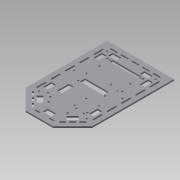
# Autodesk Inventor part: base kepala
Saved by Autodesk Inventor 2015 SP1 (Build 190203100, 203)
## iProperties
Created: 2015-02-14
Part Number: base kepala
Material: Generic
Document SubType Name: Modeling
Designer: Rafi Kurnia Putra
Density: 1 g/cm^3
Appearance: Default
Author: Rafi Kurnia Putra
Autodesk Inventor part; units mm, degrees
ref_plane "YZ Plane" through (0, 0, 0) normal (1, 0, 0) x (0, 1, 0)
ref_plane "XZ Plane" through (0, 0, 0) normal (0, 1, 0) x (-1, 0, 0)
ref_plane "XY Plane" through (0, 0, 0) normal (0, 0, 1) x (1, 0, 0)
sketch "Sketch1" plane through (0, 0, 0) normal (0, 1, 0) x (-1, 0, 0)
  line L0 (-8.75, -88.3884) -> (8.75, -88.3884)
  line L1 (-8.75, -78.3884) -> (-8.75, -88.3884)
  line L2 (8.75, -78.3884) -> (-8.75, -78.3884)
  line L3 (8.75, -88.3884) -> (8.75, -78.3884)
  line L4 (24.6113, -71.8184) -> (31.6823, -78.8894)
  line L5 (31.6823, -78.8894) -> (44.0567, -66.5151)
  line L6 (36.9856, -59.444) -> (24.6113, -71.8184)
  line L7 (44.0567, -66.5151) -> (36.9856, -59.444)
  line L8 (43.5557, -43.5826) -> (53.5557, -43.5826)
  line L9 (43.5557, -26.0826) -> (43.5557, -43.5826)
  line L10 (53.5557, -26.0826) -> (43.5557, -26.0826)
  line L11 (53.5557, -43.5826) -> (53.5557, -26.0826)
  line L12 (43.556, 62.6674) -> (53.556, 62.6674)
  line L13 (53.556, 62.6674) -> (53.556, 80.1674)
  line L14 (43.556, 80.1674) -> (43.556, 62.6674)
  line L15 (53.556, 80.1674) -> (43.556, 80.1674)
  line L16 (42.0848, 81.6386) -> (42.0848, 91.6386)
  line L17 (24.5848, 81.6386) -> (42.0848, 81.6386)
  line L18 (42.0848, 91.6386) -> (24.5848, 91.6386)
  line L19 (24.5848, 91.6386) -> (24.5848, 81.6386)
  line L20 (-24.5848, 81.6386) -> (-24.5848, 91.6386)
  line L21 (-42.0848, 81.6386) -> (-24.5848, 81.6386)
  line L22 (-42.0848, 91.6386) -> (-42.0848, 81.6386)
  line L23 (-24.5848, 91.6386) -> (-42.0848, 91.6386)
  line L24 (-53.556, 80.1674) -> (-53.556, 62.6674)
  line L25 (-43.556, 80.1674) -> (-53.556, 80.1674)
  line L26 (-43.556, 62.6674) -> (-43.556, 80.1674)
  line L27 (-53.556, 62.6674) -> (-43.556, 62.6674)
  line L28 (-43.5557, -26.0826) -> (-53.5557, -26.0826)
  line L29 (-43.5557, -43.5826) -> (-43.5557, -26.0826)
  line L30 (-53.5557, -43.5826) -> (-43.5557, -43.5826)
  line L31 (-53.5557, -26.0826) -> (-53.5557, -43.5826)
  line L32 (-32, -10.9442) -> (-32, -35.1896)
  line L33 (-22.2, -10.9442) -> (-32, -10.9442)
  line L34 (-22.2, -35.1896) -> (-22.2, -10.9442)
  line L35 (-32, -35.1896) -> (-22.2, -35.1896)
  line L36 (-31.6827, -78.8894) -> (-24.6116, -71.8184)
  line L37 (-44.057, -66.5151) -> (-31.6827, -78.8894)
  line L38 (-36.986, -59.444) -> (-44.057, -66.5151)
  line L39 (-24.6116, -71.8184) -> (-36.986, -59.444)
  line L40 (-24.5, 4.9331) -> (24.5, 4.9331)
  line L41 (24.5, 15.9376) -> (-24.5, 15.9376)
  line L42 (-24.5, 15.9376) -> (-24.5, 4.9331)
  line L43 (24.5, 4.9331) -> (24.5, 15.9376)
  circle A0 centre (-50.5965, 18.9376) radius 1.75
  circle A1 centre (-50.5965, 88.6786) radius 1.75
  circle A2 centre (-37.593, 75.6756) radius 1.75
  circle A3 centre (-32.8575, 75.4371) radius 1.75
  circle A4 centre (-32.4355, 53.6756) radius 1.75
  circle A5 centre (-32.442, 26.7171) radius 1.5
  circle A6 centre (14, 31.4596) radius 1.75
  circle A7 centre (-28, 4.9331) radius 1.75
  circle A8 centre (-49.906, -55.5042) radius 1.75
  circle A9 centre (-37.593, -48.9392) radius 1.75
  circle A10 centre (-27.94, -53.8096) radius 1.75
  circle A11 centre (-20, -65.0669) radius 1.75
  circle A12 centre (20, -65.0669) radius 1.75
  circle A13 centre (20.32, -47.4596) radius 1.75
  circle A14 centre (13.2193, -43.7996) radius 1.75
  circle A15 centre (13.2193, -19.3896) radius 1.75
  circle A16 centre (37.593, -48.9392) radius 1.75
  circle A17 centre (39.7053, -43.7996) radius 1.75
  circle A18 centre (49.9057, -55.5042) radius 1.75
  circle A19 centre (39.7053, -19.3896) radius 1.75
  circle A20 centre (28, 4.9331) radius 1.75
  circle A21 centre (32.442, 26.7171) radius 1.5
  circle A22 centre (38, 31.4596) radius 1.75
  circle A23 centre (50.5965, 18.9376) radius 1.75
  circle A24 centre (32.4485, 53.6756) radius 1.75
  circle A25 centre (32.8575, 75.4371) radius 1.75
  circle A26 centre (37.593, 75.6756) radius 1.75
  circle A27 centre (50.5965, 88.6786) radius 1.75
  line L44 (29.3575, 78.4256) -> (-29.3575, 78.4256)
  line L45 (29.3575, 72.4486) -> (29.3575, 78.4256)
  line L46 (-29.3575, 72.4486) -> (29.3575, 72.4486)
  line L47 (-29.3575, 78.4256) -> (-29.3575, 72.4486)
  line L48 (-5, -92.238) -> (5, -92.238)
  line L49 (5, -92.238) -> (5, -95.238)
  line L50 (5, -95.238) -> (-5, -95.238)
  line L51 (-5, -95.238) -> (-5, -92.238)
  line L52 (-5, -92.238) -> (5, -95.238) construction
  line L53 (5, -92.238) -> (-5, -95.238) construction
  line L54 (0, 0) -> (10, 0) construction
  line L55 (0, 0) -> (0, -10.9442) construction
  line L56 (10, -92.238) -> (20, -92.238)
  line L57 (20, -92.238) -> (20, -95.238)
  line L58 (20, -95.238) -> (10, -95.238)
  line L59 (10, -95.238) -> (10, -92.238)
  line L60 (10, -92.238) -> (20, -95.238) construction
  line L61 (20, -92.238) -> (10, -95.238) construction
  line L62 (-20, -92.238) -> (-10, -92.238)
  line L63 (-10, -92.238) -> (-10, -95.238)
  line L64 (-10, -95.238) -> (-20, -95.238)
  line L65 (-20, -95.238) -> (-20, -92.238)
  line L66 (-20, -92.238) -> (-10, -95.238) construction
  line L67 (-10, -92.238) -> (-20, -95.238) construction
  line L68 (-5, -92.238) -> (5, -92.238)
  line L69 (5, -92.238) -> (5, -95.238)
  line L70 (5, -95.238) -> (-5, -95.238)
  line L71 (-5, -95.238) -> (-5, -92.238)
  line L72 (-5, -92.238) -> (5, -95.238) construction
  line L73 (5, -92.238) -> (-5, -95.238) construction
  line L74 (39.1777, -81.0815) -> (46.2487, -74.0104)
  line L75 (46.2487, -74.0104) -> (44.1274, -71.8891)
  line L76 (44.1274, -71.8891) -> (37.0563, -78.9601)
  line L77 (37.0563, -78.9601) -> (39.1777, -81.0815)
  line L78 (39.1777, -81.0815) -> (44.1274, -71.8891) construction
  line L79 (46.2487, -74.0104) -> (37.0563, -78.9601) construction
  line L80 (0, 0) -> (-7.0711, -7.0711) construction
  line L81 (0, 0) -> (10, 0) construction
  line L82 (0, 0) -> (7.0711, -7.0711) construction
  line L83 (0, 0) -> (10, 0) construction
  line L84 (28.5711, -91.6881) -> (35.6421, -84.617)
  line L85 (35.6421, -84.617) -> (33.5208, -82.4957)
  line L86 (33.5208, -82.4957) -> (26.4497, -89.5667)
  line L87 (26.4497, -89.5667) -> (28.5711, -91.6881)
  line L88 (28.5711, -91.6881) -> (33.5208, -82.4957) construction
  line L89 (35.6421, -84.617) -> (26.4497, -89.5667) construction
  line L90 (49.7843, -70.4749) -> (56.8553, -63.4038)
  line L91 (56.8553, -63.4038) -> (54.734, -61.2825)
  line L92 (54.734, -61.2825) -> (47.6629, -68.3535)
  line L93 (47.6629, -68.3535) -> (49.7843, -70.4749)
  line L94 (49.7843, -70.4749) -> (54.734, -61.2825) construction
  line L95 (56.8553, -63.4038) -> (47.6629, -68.3535) construction
  line L96 (39.1777, -81.0815) -> (46.2487, -74.0104)
  line L97 (46.2487, -74.0104) -> (44.1274, -71.8891)
  line L98 (44.1274, -71.8891) -> (37.0563, -78.9601)
  line L99 (37.0563, -78.9601) -> (39.1777, -81.0815)
  line L100 (39.1777, -81.0815) -> (44.1274, -71.8891) construction
  line L101 (46.2487, -74.0104) -> (37.0563, -78.9601) construction
  line L102 (60.406, 8.4174) -> (57.406, 8.4174)
  line L103 (57.406, 8.4174) -> (57.406, 28.4174)
  line L104 (57.406, 28.4174) -> (60.406, 28.4174)
  line L105 (60.406, 28.4174) -> (60.406, 8.4174)
  line L106 (60.406, 8.4174) -> (57.406, 28.4174) construction
  line L107 (57.406, 8.4174) -> (60.406, 28.4174) construction
  line L108 (60.406, -21.5826) -> (57.406, -21.5826)
  line L109 (57.406, -21.5826) -> (57.406, -1.5826)
  line L110 (57.406, -1.5826) -> (60.406, -1.5826)
  line L111 (60.406, -1.5826) -> (60.406, -21.5826)
  line L112 (60.406, -21.5826) -> (57.406, -1.5826) construction
  line L113 (57.406, -21.5826) -> (60.406, -1.5826) construction
  line L114 (60.406, -51.5826) -> (57.406, -51.5826)
  line L115 (57.406, -51.5826) -> (57.406, -31.5826)
  line L116 (57.406, -31.5826) -> (60.406, -31.5826)
  line L117 (60.406, -31.5826) -> (60.406, -51.5826)
  line L118 (60.406, -51.5826) -> (57.406, -31.5826) construction
  line L119 (57.406, -51.5826) -> (60.406, -31.5826) construction
  line L120 (60.406, 38.4174) -> (57.406, 38.4174)
  line L121 (57.406, 38.4174) -> (57.406, 58.4174)
  line L122 (57.406, 58.4174) -> (60.406, 58.4174)
  line L123 (60.406, 58.4174) -> (60.406, 38.4174)
  line L124 (60.406, 38.4174) -> (57.406, 58.4174) construction
  line L125 (57.406, 38.4174) -> (60.406, 58.4174) construction
  line L126 (60.406, 8.4174) -> (57.406, 8.4174)
  line L127 (57.406, 8.4174) -> (57.406, 28.4174)
  line L128 (57.406, 28.4174) -> (60.406, 28.4174)
  line L129 (60.406, 28.4174) -> (60.406, 8.4174)
  line L130 (60.406, 8.4174) -> (57.406, 28.4174) construction
  line L131 (57.406, 8.4174) -> (60.406, 28.4174) construction
  line L132 (60.406, -21.5826) -> (57.406, -21.5826)
  line L133 (57.406, -21.5826) -> (57.406, -1.5826)
  line L134 (57.406, -1.5826) -> (60.406, -1.5826)
  line L135 (60.406, -1.5826) -> (60.406, -21.5826)
  line L136 (60.406, -21.5826) -> (57.406, -1.5826) construction
  line L137 (57.406, -21.5826) -> (60.406, -1.5826) construction
  line L138 (60.406, 68.4174) -> (57.406, 68.4174)
  line L139 (57.406, 68.4174) -> (57.406, 88.4174)
  line L140 (57.406, 88.4174) -> (60.406, 88.4174)
  line L141 (60.406, 88.4174) -> (60.406, 68.4174)
  line L142 (60.406, 68.4174) -> (57.406, 88.4174) construction
  line L143 (57.406, 68.4174) -> (60.406, 88.4174) construction
  line L144 (60.406, 38.4174) -> (57.406, 38.4174)
  line L145 (57.406, 38.4174) -> (57.406, 58.4174)
  line L146 (57.406, 58.4174) -> (60.406, 58.4174)
  line L147 (60.406, 58.4174) -> (60.406, 38.4174)
  line L148 (60.406, 38.4174) -> (57.406, 58.4174) construction
  line L149 (57.406, 38.4174) -> (60.406, 58.4174) construction
  line L150 (60.406, 8.4174) -> (57.406, 8.4174)
  line L151 (57.406, 8.4174) -> (57.406, 28.4174)
  line L152 (57.406, 28.4174) -> (60.406, 28.4174)
  line L153 (60.406, 28.4174) -> (60.406, 8.4174)
  line L154 (60.406, 8.4174) -> (57.406, 28.4174) construction
  line L155 (57.406, 8.4174) -> (60.406, 28.4174) construction
  line L156 (7.5, 95.239) -> (-7.5, 95.239)
  line L157 (-7.5, 95.239) -> (-7.5, 98.239)
  line L158 (-7.5, 98.239) -> (7.5, 98.239)
  line L159 (7.5, 98.239) -> (7.5, 95.239)
  line L160 (7.5, 95.239) -> (-7.5, 98.239) construction
  line L161 (-7.5, 95.239) -> (7.5, 98.239) construction
  line L162 (30, 95.239) -> (15, 95.239)
  line L163 (15, 95.239) -> (15, 98.239)
  line L164 (15, 98.239) -> (30, 98.239)
  line L165 (30, 98.239) -> (30, 95.239)
  line L166 (30, 95.239) -> (15, 98.239) construction
  line L167 (15, 95.239) -> (30, 98.239) construction
  line L168 (52.5, 95.239) -> (37.5, 95.239)
  line L169 (37.5, 95.239) -> (37.5, 98.239)
  line L170 (37.5, 98.239) -> (52.5, 98.239)
  line L171 (52.5, 98.239) -> (52.5, 95.239)
  line L172 (52.5, 95.239) -> (37.5, 98.239) construction
  line L173 (37.5, 95.239) -> (52.5, 98.239) construction
  line L174 (-15, 95.239) -> (-30, 95.239)
  line L175 (-30, 95.239) -> (-30, 98.239)
  line L176 (-30, 98.239) -> (-15, 98.239)
  line L177 (-15, 98.239) -> (-15, 95.239)
  line L178 (-15, 95.239) -> (-30, 98.239) construction
  line L179 (-30, 95.239) -> (-15, 98.239) construction
  line L180 (7.5, 95.239) -> (-7.5, 95.239)
  line L181 (-7.5, 95.239) -> (-7.5, 98.239)
  line L182 (-7.5, 98.239) -> (7.5, 98.239)
  line L183 (7.5, 98.239) -> (7.5, 95.239)
  line L184 (7.5, 95.239) -> (-7.5, 98.239) construction
  line L185 (-7.5, 95.239) -> (7.5, 98.239) construction
  line L186 (30, 95.239) -> (15, 95.239)
  line L187 (15, 95.239) -> (15, 98.239)
  line L188 (15, 98.239) -> (30, 98.239)
  line L189 (30, 98.239) -> (30, 95.239)
  line L190 (30, 95.239) -> (15, 98.239) construction
  line L191 (15, 95.239) -> (30, 98.239) construction
  line L192 (-37.5, 95.239) -> (-52.5, 95.239)
  line L193 (-52.5, 95.239) -> (-52.5, 98.239)
  line L194 (-52.5, 98.239) -> (-37.5, 98.239)
  line L195 (-37.5, 98.239) -> (-37.5, 95.239)
  line L196 (-37.5, 95.239) -> (-52.5, 98.239) construction
  line L197 (-52.5, 95.239) -> (-37.5, 98.239) construction
  line L198 (-15, 95.239) -> (-30, 95.239)
  line L199 (-30, 95.239) -> (-30, 98.239)
  line L200 (-30, 98.239) -> (-15, 98.239)
  line L201 (-15, 98.239) -> (-15, 95.239)
  line L202 (-15, 95.239) -> (-30, 98.239) construction
  line L203 (-30, 95.239) -> (-15, 98.239) construction
  line L204 (7.5, 95.239) -> (-7.5, 95.239)
  line L205 (-7.5, 95.239) -> (-7.5, 98.239)
  line L206 (-7.5, 98.239) -> (7.5, 98.239)
  line L207 (7.5, 98.239) -> (7.5, 95.239)
  line L208 (7.5, 95.239) -> (-7.5, 98.239) construction
  line L209 (-7.5, 95.239) -> (7.5, 98.239) construction
  line L210 (-39.1777, -81.0815) -> (-46.2487, -74.0104)
  line L211 (-46.2487, -74.0104) -> (-44.1274, -71.8891)
  line L212 (-44.1274, -71.8891) -> (-37.0563, -78.9601)
  line L213 (-37.0563, -78.9601) -> (-39.1777, -81.0815)
  line L214 (-39.1777, -81.0815) -> (-44.1274, -71.8891) construction
  line L215 (-46.2487, -74.0104) -> (-37.0563, -78.9601) construction
  line L216 (-35.6421, -84.617) -> (-33.5208, -82.4957)
  line L217 (-33.5208, -82.4957) -> (-26.4497, -89.5667)
  line L218 (-35.6421, -84.617) -> (-26.4497, -89.5667) construction
  line L219 (-28.5711, -91.6881) -> (-33.5208, -82.4957) construction
  line L220 (-28.5711, -91.6881) -> (-35.6421, -84.617)
  line L221 (-26.4497, -89.5667) -> (-28.5711, -91.6881)
  line L222 (-56.8553, -63.4038) -> (-54.734, -61.2825)
  line L223 (-54.734, -61.2825) -> (-47.6629, -68.3535)
  line L224 (-56.8553, -63.4038) -> (-47.6629, -68.3535) construction
  line L225 (-49.7843, -70.4749) -> (-54.734, -61.2825) construction
  line L226 (-49.7843, -70.4749) -> (-56.8553, -63.4038)
  line L227 (-47.6629, -68.3535) -> (-49.7843, -70.4749)
  line L228 (-46.2487, -74.0104) -> (-44.1274, -71.8891)
  line L229 (-44.1274, -71.8891) -> (-37.0563, -78.9601)
  line L230 (-46.2487, -74.0104) -> (-37.0563, -78.9601) construction
  line L231 (-39.1777, -81.0815) -> (-44.1274, -71.8891) construction
  line L232 (-39.1777, -81.0815) -> (-46.2487, -74.0104)
  line L233 (-37.0563, -78.9601) -> (-39.1777, -81.0815)
  line L234 (-60.406, 8.4174) -> (-57.406, 8.4174)
  line L235 (-57.406, 8.4174) -> (-57.406, 28.4174)
  line L236 (-57.406, 28.4174) -> (-60.406, 28.4174)
  line L237 (-60.406, 28.4174) -> (-60.406, 8.4174)
  line L238 (-60.406, 8.4174) -> (-57.406, 28.4174) construction
  line L239 (-57.406, 8.4174) -> (-60.406, 28.4174) construction
  line L240 (-57.406, -1.5826) -> (-60.406, -1.5826)
  line L241 (-60.406, -1.5826) -> (-60.406, -21.5826)
  line L242 (-60.406, -21.5826) -> (-57.406, -1.5826) construction
  line L243 (-57.406, -21.5826) -> (-60.406, -1.5826) construction
  line L244 (-60.406, -21.5826) -> (-57.406, -21.5826)
  line L245 (-57.406, -21.5826) -> (-57.406, -1.5826)
  line L246 (-57.406, -31.5826) -> (-60.406, -31.5826)
  line L247 (-60.406, -31.5826) -> (-60.406, -51.5826)
  line L248 (-60.406, -51.5826) -> (-57.406, -31.5826) construction
  line L249 (-57.406, -51.5826) -> (-60.406, -31.5826) construction
  line L250 (-60.406, -51.5826) -> (-57.406, -51.5826)
  line L251 (-57.406, -51.5826) -> (-57.406, -31.5826)
  line L252 (-57.406, 58.4174) -> (-60.406, 58.4174)
  line L253 (-60.406, 58.4174) -> (-60.406, 38.4174)
  line L254 (-60.406, 38.4174) -> (-57.406, 58.4174) construction
  line L255 (-57.406, 38.4174) -> (-60.406, 58.4174) construction
  line L256 (-60.406, 38.4174) -> (-57.406, 38.4174)
  line L257 (-57.406, 38.4174) -> (-57.406, 58.4174)
  line L258 (-57.406, 28.4174) -> (-60.406, 28.4174)
  line L259 (-60.406, 28.4174) -> (-60.406, 8.4174)
  line L260 (-60.406, 8.4174) -> (-57.406, 28.4174) construction
  line L261 (-57.406, 8.4174) -> (-60.406, 28.4174) construction
  line L262 (-60.406, 8.4174) -> (-57.406, 8.4174)
  line L263 (-57.406, 8.4174) -> (-57.406, 28.4174)
  line L264 (-57.406, -1.5826) -> (-60.406, -1.5826)
  line L265 (-60.406, -1.5826) -> (-60.406, -21.5826)
  line L266 (-60.406, -21.5826) -> (-57.406, -1.5826) construction
  line L267 (-57.406, -21.5826) -> (-60.406, -1.5826) construction
  line L268 (-60.406, -21.5826) -> (-57.406, -21.5826)
  line L269 (-57.406, -21.5826) -> (-57.406, -1.5826)
  line L270 (-57.406, 88.4174) -> (-60.406, 88.4174)
  line L271 (-60.406, 88.4174) -> (-60.406, 68.4174)
  line L272 (-60.406, 68.4174) -> (-57.406, 88.4174) construction
  line L273 (-57.406, 68.4174) -> (-60.406, 88.4174) construction
  line L274 (-60.406, 68.4174) -> (-57.406, 68.4174)
  line L275 (-57.406, 68.4174) -> (-57.406, 88.4174)
  line L276 (-57.406, 58.4174) -> (-60.406, 58.4174)
  line L277 (-60.406, 58.4174) -> (-60.406, 38.4174)
  line L278 (-60.406, 38.4174) -> (-57.406, 58.4174) construction
  line L279 (-57.406, 38.4174) -> (-60.406, 58.4174) construction
  line L280 (-60.406, 38.4174) -> (-57.406, 38.4174)
  line L281 (-57.406, 38.4174) -> (-57.406, 58.4174)
  line L282 (-57.406, 28.4174) -> (-60.406, 28.4174)
  line L283 (-60.406, 28.4174) -> (-60.406, 8.4174)
  line L284 (-60.406, 8.4174) -> (-57.406, 28.4174) construction
  line L285 (-57.406, 8.4174) -> (-60.406, 28.4174) construction
  line L286 (-60.406, 8.4174) -> (-57.406, 8.4174)
  line L287 (-57.406, 8.4174) -> (-57.406, 28.4174)
  line L288 (70, 107.8327) -> (-70.0003, 107.8327)
  line L289 (-70.0003, 107.8327) -> (-70.0003, -63.8276)
  line L290 (-70.0003, -63.8276) -> (-28.9952, -104.8327)
  line L291 (-28.9952, -104.8327) -> (28.9948, -104.8327)
  line L292 (28.9948, -104.8327) -> (70, -63.8276)
  line L293 (70, -63.8276) -> (70, 107.8327)
  point P0 (0, -93.738)
  point P1 (15, -93.738)
  point P2 (-15, -93.738)
  point P3 (0, -93.738)
  point P4 (42.7132, -77.5459)
  point P5 (37.8695, -72.7022)
  point P6 (41.6525, -76.4853)
  point P7 (32.1066, -88.1525)
  point P8 (27.2629, -83.3088)
  point P9 (31.0459, -87.0919)
  point P10 (53.3198, -66.9393)
  point P11 (48.4761, -62.0956)
  point P12 (52.2591, -65.8787)
  point P13 (42.7132, -77.5459)
  point P14 (37.8695, -72.7022)
  point P15 (41.6525, -76.4853)
  point P16 (60.4057, 18.4174)
  point P17 (58.906, 18.4174)
  point P18 (60.4057, -11.5826)
  point P19 (58.906, -11.5826)
  point P20 (60.4057, -41.5826)
  point P21 (58.906, -41.5826)
  point P22 (60.4057, 48.4174)
  point P23 (58.906, 48.4174)
  point P24 (60.4057, 18.4174)
  point P25 (58.906, 18.4174)
  point P26 (60.4057, -11.5826)
  point P27 (58.906, -11.5826)
  point P28 (60.4057, 78.4174)
  point P29 (58.906, 78.4174)
  point P30 (60.4057, 48.4174)
  point P31 (58.906, 48.4174)
  point P32 (60.4057, 18.4174)
  point P33 (58.906, 18.4174)
  point P34 (0, 96.739)
  point P35 (0, 96.739)
  point P36 (22.5, 96.739)
  point P37 (22.5, 96.739)
  point P38 (45, 96.739)
  point P39 (45, 96.739)
  point P40 (-22.5, 96.739)
  point P41 (-22.5, 96.739)
  point P42 (0, 96.739)
  point P43 (0, 96.739)
  point P44 (22.5, 96.739)
  point P45 (22.5, 96.739)
  point P46 (-45, 96.739)
  point P47 (-45, 96.739)
  point P48 (-22.5, 96.739)
  point P49 (-22.5, 96.739)
  point P50 (0, 96.739)
  point P51 (0, 96.739)
  point P52 (-42.7132, -77.5459)
  point P53 (-41.6525, -76.4853)
  point P54 (-31.0459, -87.0919)
  point P55 (-27.2629, -83.3088)
  point P56 (-32.1066, -88.1525)
  point P57 (-52.2591, -65.8787)
  point P58 (-53.3198, -66.9393)
  point P59 (-41.6525, -76.4853)
  point P60 (-37.8695, -72.7022)
  point P61 (-42.7132, -77.5459)
  point P62 (-58.906, 18.4174)
  point P63 (-58.906, -11.5826)
  point P64 (-58.906, -41.5826)
  point P65 (-58.906, 48.4174)
  point P66 (-58.906, 18.4174)
  point P67 (-58.906, -11.5826)
  point P68 (-58.906, 78.4174)
  point P69 (-58.906, 48.4174)
  point P70 (-58.906, 18.4174)
  dimension "d0" = 10
  dimension "d1" = 3
  dimension "d4" = 15
  dimension "d7" = 15
  dimension "d10" = 1.5
  dimension "d11" = 10
  dimension "d12" = 3
  dimension "d13" = 10
  dimension "d14" = 135
  dimension "d15" = 45
  dimension "d18" = 15
  dimension "d21" = 15
  dimension "d24" = 3
  dimension "d25" = 20
  dimension "d28" = 30
  dimension "d31" = 30
  dimension "d34" = 15
  dimension "d35" = 3
  dimension "d38" = 22.5
  dimension "d41" = 22.5
  dimension "d49" = 76.8216
  constraints: 588 end point, 80 midpoint, 71 symmetric about line, 28 centre point, 10 horizontal, 9 parallel, 4 perpendicular, 3 vertical, 2 equal length, 269 other
  measures "d0" distance of L49.end L50.end
  measures "d1" distance of L48.end L49.end
  measures "d4" distance of L48.start L59.end
  measures "d7" distance of L48.start L65.end
  measures "d10" distance of point (41.653, -76.485) point (42.713, -77.546)
  measures "d11" distance of L74.start L74.end
  measures "d12" distance of L75.end L74.end
  measures "d13" distance of L54.start L80.end
  measures "d14" angle of L80 L81
  measures "d15" angle of L82 L83
  measures "d18" distance of L75.end L85.end
  measures "d21" distance of L75.end L91.end
  measures "d24" distance of L103.end L104.end
  measures "d25" distance of L102.end L103.end
  measures "d28" distance of L104.end L110.end
  measures "d31" distance of L104.end L122.end
  measures "d34" distance of L157.end L158.end
  measures "d35" distance of L156.end L157.end
  measures "d38" distance of L156.end L163.start
  measures "d41" distance of L156.end L175.start
  measures "d49" distance from line of point (60.406, 18.417) L168
extrude "Extrusion2" add sketch "Sketch1" along normal blind 3 contours L48 L49 L50 L51 | L293 L292 L291 L290 L289 L288
body "Solid2"
